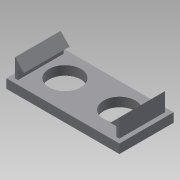
# Autodesk Inventor part: Part1
Saved by Autodesk Inventor 2015 SP1 (Build 190203100, 203)
## iProperties
Created: 2015-03-28
Part Number: Part1
Material: Generic
Document SubType Name: Modeling
Designer: Rafi Kurnia Putra
Density: 1 g/cm^3
Appearance: Default
Author: Rafi Kurnia Putra
Autodesk Inventor part; units mm, degrees
ref_plane "YZ Plane" through (0, 0, 0) normal (1, 0, 0) x (0, 1, 0)
ref_plane "XZ Plane" through (0, 0, 0) normal (0, 1, 0) x (-1, 0, 0)
ref_plane "XY Plane" through (0, 0, 0) normal (0, 0, 1) x (1, 0, 0)
sketch "Sketch1" plane through (0, 0, 0) normal (0, 0, 1) x (1, 0, 0)
  circle A0 centre (-9, 0) radius 5.25
  circle A1 centre (9, 0) radius 5.25
  line L0 (-16.175, 6.75) -> (16.175, 6.75)
  line L1 (-16.175, -8.25) -> (-16.175, 6.75)
  line L2 (16.175, -8.25) -> (-16.175, -8.25)
  line L3 (16.175, 6.75) -> (16.175, -8.25)
  line L4 (-16.175, 6.75) -> (16.175, -8.25) construction
  line L5 (16.175, 6.75) -> (-16.175, -8.25) construction
  point P0 (0, 0)
  point P1 (0, -7.6531)
  point P2 (14.6494, -5.75)
  point P3 (0, -0.75)
  dimension "d2" = 10.5
  dimension "d3" = 32.35
  dimension "d4" = 32.35
  dimension "d5" = 16.175
  dimension "d6" = 15
  dimension "d7" = 15
  dimension "d8" = 12.5
  dimension "d9" = 18
  dimension "d12" = 9
  dimension "d13" = 9
  dimension "d14" = 10.5
  dimension "d15" = 6.75
  dimension "d16" = 6.75
  constraints: 12 end point, 2 centre point, 1 midpoint, 1 other
  measures "d2" diameter of A0
  measures "d3" distance of L0.start L0.end
  measures "d4" distance of L2.start L1.start
  measures "d5" distance from line of L1 point (0, -7.653)
  measures "d6" distance of L0.end L2.start
  measures "d7" distance of L1.start L0.start
  measures "d8" distance from line of point (14.649, -5.75) L0
  measures "d9" distance of A1.centre A0.centre
  measures "d12" distance of point (0, 0) A0.centre
  measures "d13" distance of point (0, 0) A1.centre
  measures "d14" diameter of A1
  measures "d15" distance from line of point (0, 0) L0
  measures "d16" vertical distance of point (0, 0) L0.start
extrude "Extrusion1" add sketch "Sketch1" along normal blind 3
sketch "Sketch2" plane through (0, 0, 0) normal (0, 0, -1) x (-1, 0, 0)
  circle A0 centre (-9, 0) radius 5.25 projected
  circle A1 centre (9, 0) radius 5.25 projected
  line L0 (-16.175, 6.75) -> (16.175, 6.75) projected
  line L1 (-16.175, -8.25) -> (-16.175, 6.75) projected
  line L2 (16.175, -8.25) -> (-16.175, -8.25) projected
  line L3 (16.175, 6.75) -> (16.175, -8.25) projected
  line L4 (-16.175, 6.75) -> (-17.175, 6.75)
  line L5 (-17.175, 6.75) -> (-17.175, -8.25)
  line L6 (-17.175, -8.25) -> (-16.175, -8.25)
  line L7 (-16.175, -8.25) -> (-16.175, 6.75)
  line L8 (16.175, 6.75) -> (17.175, 6.75)
  line L9 (17.175, 6.75) -> (17.175, -8.25)
  line L10 (17.175, -8.25) -> (16.175, -8.25)
  line L11 (16.175, -8.25) -> (16.175, 6.75)
  point P0 (0, 0)
  dimension "d17" = 1
  dimension "d18" = 1
  constraints: 16 end point, 4 parallel, 2 horizontal, 2 perpendicular, 1 point on line
  measures "d17" distance of L6.end L5.end
  measures "d18" distance of L9.end L10.end
extrude "Extrusion2" add sketch "Sketch2" against normal blind 6 contours L1 L6 L5 L4 | L8 L9 L10 L3
sketch "Sketch3" plane through (-17.175, -8.25, 0) normal (0, -1, 0) x (1, 0, 0)
  line L0 (0, 6) -> (3, 6)
  line L1 (3, 6) -> (0, 9)
  line L2 (0, 9) -> (0, 6)
  line L3 (34.35, 6) -> (31.35, 6)
  line L4 (34.35, 6) -> (33.35, 6) projected
  line L5 (31.35, 6) -> (34.35, 9)
  line L6 (34.35, 9) -> (34.35, 6)
  point P0 (17.175, 0)
  dimension "d21" = 45
  dimension "d22" = 3
  dimension "d23" = 45
  dimension "d35" = 3
  constraints: 12 end point, 2 perpendicular, 1 collinear, 1 horizontal
  measures "d21" angle of L1 L0
  measures "d22" distance of L3.start L3.end
  measures "d23" angle of L3 L5
  measures "d35" distance of L0.start L0.end
extrude "Extrusion3" add sketch "Sketch3" against normal blind 15
sketch "Sketch4" plane through (0, 0, 0) normal (0, 0, -1) x (-1, 0, 0)
  circle A0 centre (-9, 0) radius 5.25 projected
  circle A1 centre (9, 0) radius 5.25 projected
  line L0 (-17.175, 6.75) -> (17.175, 6.75) projected
  line L1 (-17.175, 6.75) -> (-17.175, -8.25) projected
  line L2 (-17.175, -8.25) -> (17.175, -8.25) projected
  line L3 (17.175, -8.25) -> (17.175, 6.75) projected
  line L4 (17.175, -8.25) -> (18.5892, -9.6642)
  line L5 (17.175, -8.25) -> (19.175, -8.25) construction
  line L6 (17.175, 6.75) -> (18.5892, 8.1642)
  line L7 (17.175, 6.75) -> (19.175, 6.75) construction
  line L8 (-17.175, 6.75) -> (-18.5892, 8.1642)
  line L9 (-17.175, 6.75) -> (-15.175, 6.75) construction
  line L10 (-17.175, 6.75) -> (-17.175, -8.25) projected
  line L11 (-18.5892, 8.1642) -> (18.5892, 8.1642)
  line L12 (18.5892, -9.6642) -> (18.5892, 8.1642)
  line L13 (18.5892, -9.6642) -> (-18.5892, -9.6642)
  line L14 (18.5892, -9.6642) -> (55.7676, -9.6642) construction
  line L15 (-18.5892, -9.6642) -> (-18.5892, 8.1642)
  point P0 (0, 0)
  dimension "d26" = 2
  dimension "d27" = 45
  dimension "d28" = 2
  dimension "d29" = 45
  dimension "d30" = 2
  dimension "d31" = 135
  dimension "d32" = 180
  constraints: 22 end point, 4 equal length, 4 horizontal, 1 perpendicular
  measures "d26" distance of L2.end L4.end
  measures "d27" angle of L4 L5
  measures "d28" distance of L0.end L6.end
  measures "d29" angle of L7 L6
  measures "d30" distance of L0.start L8.end
  measures "d31" angle of L9 L8
  measures "d32" angle of L13 L14
extrude "Extrusion4" add sketch "Sketch4" against normal blind 3 contours L8 L11 L6 L0 | L1 L2 L4 L13 L15 L8 | L6 L12 L4 L3
equation "\"d4\" = d3"
equation "\"d5\" = 0.5 * d4"
equation "\"d7\" = d6"
equation "\"d12\" = 0.5 * d9"
equation "\"d13\" = d12"
equation "\"d14\" = d2"
equation "\"d16\" = d15"
body "Solid1"
